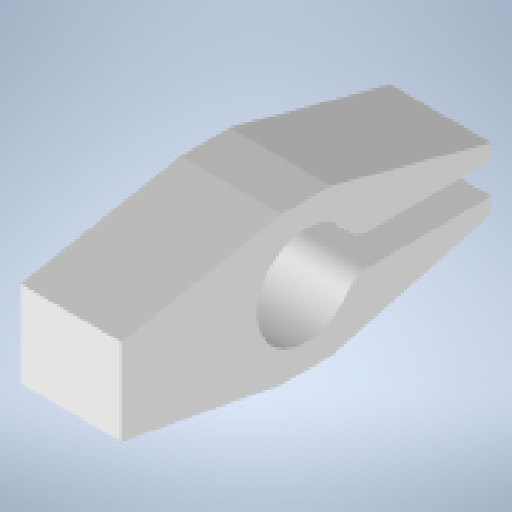
# Autodesk Inventor part: BeltClampM5
Saved by Autodesk Inventor 2023 (Build 270158000, 158)
## iProperties
Created: 2023-09-08
Part Number: BeltClampM5
Material: Generic
Document SubType Name: Modeling
Designer: Felix
Density: 1 g/cm^3
Appearance: Default
Author: Felix
Autodesk Inventor part; units mm, degrees
ref_plane "YZ Plane" through (0, 0, 0) normal (1, 0, 0) x (0, 1, 0)
ref_plane "XZ Plane" through (0, 0, 0) normal (0, 1, 0) x (-1, 0, 0)
ref_plane "XY Plane" through (0, 0, 0) normal (0, 0, 1) x (1, 0, 0)
sketch "Sketch1" plane through (0, 0, 0) normal (1, 0, 0) x (0, 1, 0)
  line L0 (0, 0) -> (0, 15.0436) construction
  line L1 (-1.25, 0) -> (-1.25, 10)
  line L2 (1.25, 0) -> (1.25, 10)
  circle A0 centre (0, 15.0436) radius 2
  arc A1 (2.1667, 11.6812) -> (-2.1667, 11.6812) centre (0, 15.0436) ccw
  arc A2 (-1.25, 10) -> (-2.1667, 11.6812) centre (-3.25, 10) ccw
  arc A3 (2.1667, 11.6812) -> (1.25, 10) centre (3.25, 10) ccw
  line L3 (2.5, 20.0436) -> (-2.5, 20.0436) construction
  line L4 (-2.5, 20.0436) -> (-2.5, 30.0436) construction
  line L5 (-2.5, 30.0436) -> (2.5, 30.0436) construction
  line L6 (2.5, 30.0436) -> (2.5, 20.0436) construction
  line L7 (-6, 0) -> (6, 0)
  line L8 (6, 0) -> (6, 30.0436)
  line L9 (6, 30.0436) -> (-6, 30.0436)
  line L10 (-6, 30.0436) -> (-6, 0)
  line L11 (2.5, 0) -> (6, 13.0436)
  line L12 (6, 17.0436) -> (3.5, 30.0436)
  line L13 (6, 13.0436) -> (-6.1446, 13.0436) construction
  line L14 (6, 17.0436) -> (-6.1446, 17.0436) construction
  line L15 (-2.5, 0) -> (-6, 13.0436)
  line L16 (-6, 17.0436) -> (-3.5, 30.0436)
  point P0 (0, 20.0436)
  dimension "d0" = 2.5
  dimension "d1" = 4
  dimension "d2" = 2
  dimension "d3" = 2
  dimension "d4" = 10
  dimension "d5" = 10
  dimension "d6" = 5
  dimension "d7" = 1
  dimension "d8" = 2
  dimension "d9" = 2
  dimension "d10" = 7
  constraints: 34 end point, 6 parallel, 6 point on circle, 6 point on line, 6 tangent, 4 centre point, 4 perpendicular, 4 symmetric about line, 2 horizontal, 2 horizontal alignment, 2 midpoint, 1 coincident, 1 vertical, 1 vertical alignment, 2 other
  measures "d0" distance between parallel lines of L2 L1
  measures "d1" diameter of A0
  measures "d2" radial gap between concentric circles of A0 A1
  measures "d3" radius of A3
  measures "d4" distance of L2.start L2.end
  measures "d5" distance of L3.end L4.end
  measures "d6" distance of L4.end L5.end
  measures "d7" distance edge to line of A1 L3
  measures "d8" distance edge to line of A1 L8
  measures "d9" distance edge to line of A1 L10
  measures "d10" distance of L16.end L12.end
extrude "Extrusion1" add sketch "Sketch1" along normal blind 7.2 contours L7 L15 L10 L16 L9 L12 L8 L11 L2 A3 A1 A2 L1
sketch "Sketch2" plane through (0, 0, 0) normal (-1, 0, 0) x (0, 0, 1)
  line L0 (0, -2.5) -> (0, -1.25) projected
  line L1 (0, 1.25) -> (0, 2.5) projected
  line L2 (0, 2.5) -> (13.0436, 6) projected
  line L3 (13.0436, 6) -> (17.0436, 6) projected
  line L4 (17.0436, 6) -> (30.0436, 3.5) projected
  line L5 (30.0436, 3.5) -> (30.0436, -3.5) projected
  line L6 (30.0436, -3.5) -> (17.0436, -6) projected
  line L7 (17.0436, -6) -> (13.0436, -6) projected
  line L8 (13.0436, -6) -> (0, -2.5) projected
  line L9 (0, -2.5) -> (0, -1.25) projected
  line L10 (0, 1.25) -> (0, -1.25)
  point P0 (0, 0)
  constraints: 2 end point, 1 vertical
extrude "Extrusion2" add sketch "Sketch2" along normal blind 2
sketch "Sketch3" plane through (-2, 0, 0) normal (-1, 0, 0) x (0, 0, 1)
  arc A0 (11.6812, -2.1667) -> (11.6812, 2.1667) centre (15.0436, 0) ccw projected
  point P0 (0, 0)
hole "Hole1" at (-2, 0, 15.0436) direction (1, 0, 0) diameter 3.4 end through all countersink diameter 6.3 countersink angle 90 clearance for "Countersunk Flat Head Screw DIN EN ISO 2009" size "M3" standard "DIN"
sketch "Sketch4" plane through (7.2, -3.5, 30.0436) normal (0, 0, 1) x (1, 0, 0)
  line L0 (-9.2, 0) -> (0, 0) construction
  line L1 (0, 7) -> (0, 0) construction
  line L2 (-9.2, 7) -> (0, 7) construction
  line L3 (-9.2, 0) -> (-9.2, 7) construction
  line L4 (0, 7) -> (-9.2, 0) construction
  line L5 (-9.2, 7) -> (0, 0) construction
  point P0 (-7.2, 3.5)
  point P1 (-4.6, 3.5)
  constraints: 4 end point, 1 midpoint
hole "Hole2" at (2.6, 0, 30.0436) direction (0, 0, -1) diameter 5 depth 10
equation "\"d9\" = d8"
body "Solid1"
